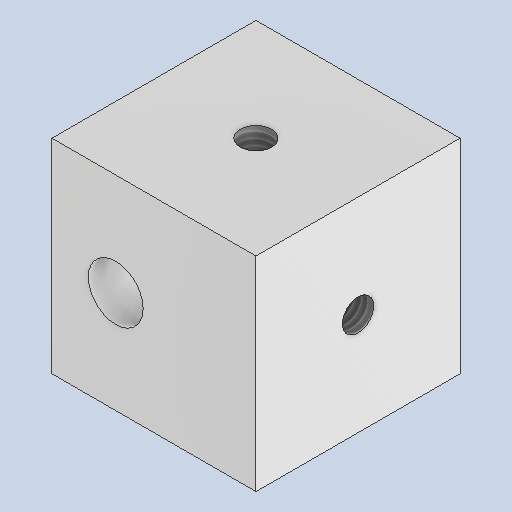
# Autodesk Inventor part: Frameblock
Saved by Autodesk Inventor 2025 (Build 290162010, 162A)
## iProperties
Created: 2025-01-27
Part Number: Frameblock
Material: PC/ABS-Kunststoff, 3DDruck, PLA
Document SubType Name: Modeling
Designer: Admin
Density: 1.1 g/cm^3
Appearance: Glatt - Weiß(2)
Author: Admin
Autodesk Inventor part; units mm, degrees
ref_plane "YZ Plane" through (0, 0, 0) normal (1, 0, 0) x (0, 1, 0)
ref_plane "XZ Plane" through (0, 0, 0) normal (0, 1, 0) x (-1, 0, 0)
ref_plane "XY Plane" through (0, 0, 0) normal (0, 0, 1) x (1, 0, 0)
sketch "Skizze1" plane through (0, 0, 0) normal (1, 0, 0) x (0, 1, 0)
  line L0 (0, 0) -> (16, 0)
  line L1 (16, 0) -> (16, -16)
  line L2 (16, -16) -> (0, -16)
  line L3 (0, -16) -> (0, 0)
  dimension "d0" = 16
  dimension "d1" = 16
  constraints: 8 end point, 2 parallel, 1 horizontal, 1 perpendicular
  measures "d0" distance of L1.end L2.end
  measures "d1" distance of L0.end L1.end
extrude "Extrusion1" add sketch "Skizze1" along normal blind 16
sketch "Skizze2" plane through (0, 16, 0) normal (0, 1, 0) x (1, 0, 0)
  line L0 (5, 8) -> (0, 8)
  line L1 (0, 16) -> (0, 0) projected
  dimension "d4" = 5
  constraints: 2 end point, 1 midpoint, 1 perpendicular
  measures "d4" distance of L0.start L0.end
hole "Bohrung1" at (5, 16, -8) direction (0, -1, 0) diameter 4.3 end through all countersink diameter 11 countersink angle 90 clearance for "Flachkopfmaschinenschraube" size "M4" standard "ANSI Metrisches M Profil"
sketch "Skizze3" plane through (0, 0, 0) normal (0, 0, 1) x (1, 0, 0)
  line L0 (0, 16) -> (0, 0) projected
  line L1 (0, 8) -> (8, 8)
  dimension "d12" = 8
  constraints: 2 end point, 1 coincident, 1 midpoint, 1 perpendicular
  measures "d12" distance of L1.start L1.end
hole "Bohrung2" at (8, 8, 0) direction (0, 0, -1) diameter 2.459 end through all thread size "M3x0.5" class "6H" standard "ANSI Metric M Profile"
sketch "Skizze4" plane through (16, 0, 0) normal (1, 0, 0) x (0, 0, -1)
  line L0 (10.15, 0) -> (5.85, 0) projected
  line L1 (8, 0) -> (8, 8)
  point P0 (0, 0)
  dimension "d20" = 8
  constraints: 2 end point, 1 midpoint, 1 vertical
  measures "d20" distance of L1.start L1.end
hole "Bohrung3" at (16, 8, -8) direction (-1, 0, 0) diameter 2.459 end through all thread size "M3x0.5" class "6H" standard "ANSI Metric M Profile"
